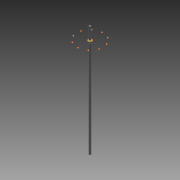
# Autodesk Inventor part: Worm Gear
Saved by Autodesk Inventor 2011 (Build 150239000, 239)
## iProperties
Created: 2011-11-28
Part Number: Worm Gear
Material: Steel, Mild
Document SubType Name: Modeling
Designer: Tom
Categories: <?xml version="1.0" encoding="UTF-16"?> <MemberInstance><Categories><FamilyTemplate><FamilyTemplateParameter ValueType="xs:double" Id="1" ObjectReferenceKey="da_z" ObjectType="kUserParameterObject"/><FamilyTemplateParameter ValueType="xs:double" Id="2" ObjectReferenceKey="da_b" ObjectType="kUserParameterObject"/><FamilyTemplateParameter ValueType="xs:double" Id="3" ObjectReferenceKey="da_beta" ObjectType="kUserParameterObject"/><FamilyTemplateParameter ValueType="xs:double" Id="4" ObjectReferenceKey="da_m" ObjectType="kUserParameterObject"/><FamilyTemplateParameter ValueType="xs:double" Id="5" ObjectReferenceKey="da_alpha" ObjectType="kUserParameterObject"/><FamilyTemplateParameter ValueType="xs:double" Id="6" ObjectReferenceKey="da_da" ObjectType="kUserParameterObject"/><FamilyTemplateParameter ValueType="xs:double" Id="7" ObjectReferenceKey="da_aw" ObjectType="kUserParameterObject"/><FamilyTemplateParameter ValueType="xs:double" Id="8" ObjectReferenceKey="da_px" ObjectType="kUserParameterObject"/><FamilyTemplateParameter ValueType="xs:double" Id="9" ObjectReferenceKey="da_d" ObjectType="kUserParameterObject"/><FamilyTemplateParameter ValueType="xs:double" Id="10" ObjectReferenceKey="da_dae" ObjectType="kUserParameterObject"/><FamilyTemplateParameter ValueType="xs:double" Id="11" ObjectReferenceKey="da_fi" ObjectType="kUserParameterObject"/><FamilyTemplateParameter ValueType="xs:string" Id="12" ObjectReferenceKey="EAIAABAAAAAWFwAAAAAAAIAAAAAAAAAA" ObjectType="83910656" SubObjectId="SurfaceGeometry"/></FamilyTemplate><ParamToTemplateMap><ParamToTemplate CategoryParameter="//CategoryParameter[@InternalName='046C89C9-8512-4d59-83FE-43B91F4F132A']" TemplateParameter="1"/><ParamToTemplate CategoryParameter="//CategoryParameter[@InternalName='2552DF32-E462-4b46-AEBF-C6C7768E72AC']" TemplateParameter="2"/><ParamToTemplate CategoryParameter="//CategoryParameter[@InternalName='C9EE641D-15FC-4fae-A226-E94C4372FDD7']" TemplateParameter="3"/><ParamToTemplate><ParamToTemplate CategoryParameter="//CategoryParameter[@InternalName='00B6519A-459B-49c7-AD84-2E56D39A5744']" ConstantValue="0.000000"/></ParamToTemplate><ParamToTemplate><ParamToTemplate CategoryParameter="//CategoryParameter[@InternalName='04B31F0E-C7A6-4894-AA32-9629BEFACF47']" ConstantValue="1.000000"/></ParamToTemplate><ParamToTemplate><ParamToTemplate CategoryParameter="//CategoryParameter[@InternalName='43CBEC2E-7847-49e7-A936-2F7889FCB2D9']" ConstantValue="0.200000"/></ParamToTemplate><ParamToTemplate><ParamToTemplate CategoryParameter="//CategoryParameter[@InternalName='B1EFC894-105D-4ebd-86BF-FA20ED196853']" ConstantValue="0.300000"/></ParamToTemplate><ParamToTemplate><ParamToTemplate CategoryParameter="//CategoryParameter[@InternalName='51175063-3D10-4879-93E8-6246FE8B403D']" ConstantValue="2060000000.000000"/></ParamToTemplate><ParamToTemplate><ParamToTemplate CategoryParameter="//CategoryParameter[@InternalName='A3A52E27-4454-46a9-B0BD-C932399B70AF']" ConstantValue="0.300000"/></ParamToTemplate><ParamToTemplate CategoryParameter="//CategoryParameter[@InternalName='91B76062-C214-41d9-B1B9-14D2AB99603D']" TemplateParameter="4"/><ParamToTemplate CategoryParameter="//CategoryParameter[@InternalName='2D373A89-B862-43d6-8D0B-0CBF12AB9F6C']" TemplateParameter="5"/><ParamToTemplate CategoryParameter="//CategoryParameter[@InternalName='37777632-D6A2-4fac-9D53-DB8ACD95C989']" TemplateParameter="6"/><ParamToTemplate CategoryParameter="//CategoryParameter[@InternalName='FD1017F1-B727-4f7e-9707-0F86F1FF9423']" TemplateParameter="7"/><ParamToTemplate CategoryParameter="//CategoryParameter[@InternalName='3BF567DA-17EF-48d8-80EA-D119B07F6463']" TemplateParameter="8"/><ParamToTemplate CategoryParameter="//CategoryParameter[@InternalName='BF5A1E7E-5373-4a22-AAD3-F583781FCF3C']" TemplateParameter="9"/><ParamToTemplate CategoryParameter="//CategoryParameter[@InternalName='2A200944-5A8C-41ca-B96E-8520D2E510F1']" TemplateParameter="10"/><ParamToTemplate CategoryParameter="//CategoryParameter[@InternalName='E77AC4FD-7B43-4566-B0ED-7CA70B976BC8']" TemplateParameter="11"/><ParamToTemplate><ParamToTemplate CategoryParameter="//CategoryParameter[@InternalName='D4F72237-D604-435a-AD0B-F738B7463A00']" ConstantValue="110.000000"/></ParamToTemplate><ParamToTemplate><ParamToTemplate CategoryParameter="//CategoryParameter[@InternalName='9E1B4470-B2D3-4ff1-B813-535BB4CDF51A']" ConstantValue="2000000.000000"/></ParamToTemplate><ParamToTemplate><ParamToTemplate CategoryParameter="//CategoryParameter[@InternalName='A7A89E9A-52E6-4d4f-86CF-A81914F22AA4']" ConstantValue="250000000.000000"/></ParamToTemplate><ParamToTemplate><ParamToTemplate CategoryParameter="//CategoryParameter[@InternalName='B02FABAC-469F-4ad8-A219-DB4578299DF6']" ConstantValue="250000000.000000"/></ParamToTemplate><ParamToTemplate><ParamToTemplate CategoryParameter="//CategoryParameter[@InternalName='E6981962-40D5-4343-A0AD-C263FCC47E10']" ConstantValue="9.000000"/></ParamToTemplate><ParamToTemplate><ParamToTemplate CategoryParameter="//CategoryParameter[@InternalName='B958E99F-2BCD-4955-8634-793EB7B37B89']" ConstantValue="8.000000"/></ParamToTemplate><ParamToTemplate><ParamToTemplate CategoryParameter="//CategoryParameter[@InternalName='4AD49A87-569D-440f-A541-E3B52A6A9DCE']" ConstantValue="1200.000000"/></ParamToTemplate><ParamToTemplate><ParamToTemplate CategoryParameter="//CategoryParameter[@InternalName='4E5813A0-330D-4b41-BE23-D880B01A1D55']" ConstantValue="1650000.000000"/></ParamToTemplate><ParamToTemplate><ParamToTemplate CategoryParameter="//CategoryParameter[@InternalName='19EB8C86-AA88-4253-B4AA-2F5DF1CE171A']" ConstantValue="6000.000000"/></ParamToTemplate><ParamToTemplate CategoryParameter="//CategoryParameter[@InternalName='27C3BAF2-7550-4e4b-AE2C-0DB134B7D9B7']" TemplateParameter="12"/></ParamToTemplateMap><Category DisplayName="Gear" InternalName="DC85795E-93AB-48d5-8EEE-5A27447B64BD" Mnemonic="Gear"><CategoryParameter DisplayName="z" InternalName="046C89C9-8512-4d59-83FE-43B91F4F132A" Mnemonic="z"/><CategoryParameter DisplayName="b|.2|" InternalName="2552DF32-E462-4b46-AEBF-C6C7768E72AC" Mnemonic="b"/><CategoryParameter DisplayName="||b|" InternalName="C9EE641D-15FC-4fae-A226-E94C4372FDD7" Mnemonic="beta"/><CategoryParameter DisplayName="x" InternalName="00B6519A-459B-49c7-AD84-2E56D39A5744" Mnemonic="x"/><CategoryParameter DisplayName="a*" InternalName="04B31F0E-C7A6-4894-AA32-9629BEFACF47" Mnemonic="a"/><CategoryParameter DisplayName="c*" InternalName="43CBEC2E-7847-49e7-A936-2F7889FCB2D9" Mnemonic="c"/><CategoryParameter DisplayName="r|.f|*" InternalName="B1EFC894-105D-4ebd-86BF-FA20ED196853" Mnemonic="rf"/><CategoryParameter DisplayName="E" InternalName="51175063-3D10-4879-93E8-6246FE8B403D" Mnemonic="E"/><CategoryParameter DisplayName="||m|" InternalName="A3A52E27-4454-46a9-B0BD-C932399B70AF" Mnemonic="mi"/><Category DisplayName="WormGear" InternalName="1B25C7EF-093B-4025-B3D3-619CD2A4550C" Mnemonic="WormGear"><CategoryParameter DisplayName="m" InternalName="91B76062-C214-41d9-B1B9-14D2AB99603D" Mnemonic="m"/><CategoryParameter DisplayName="||a|" InternalName="2D373A89-B862-43d6-8D0B-0CBF12AB9F6C" Mnemonic="alpha"/><CategoryParameter DisplayName="d|.a|" InternalName="37777632-D6A2-4fac-9D53-DB8ACD95C989" Mnemonic="da"/><CategoryParameter DisplayName="a|.w|" InternalName="FD1017F1-B727-4f7e-9707-0F86F1FF9423" Mnemonic="aw"/><CategoryParameter DisplayName="p|.x|" InternalName="3BF567DA-17EF-48d8-80EA-D119B07F6463" Mnemonic="px"/><CategoryParameter DisplayName="d" InternalName="BF5A1E7E-5373-4a22-AAD3-F583781FCF3C" Mnemonic="d"/><CategoryParameter DisplayName="dae" InternalName="2A200944-5A8C-41ca-B96E-8520D2E510F1" Mnemonic="dae"/><CategoryParameter DisplayName="||d|" InternalName="E77AC4FD-7B43-4566-B0ED-7CA70B976BC8" Mnemonic="fi"/><CategoryParameter DisplayName="VHV" InternalName="D4F72237-D604-435a-AD0B-F738B7463A00" Mnemonic="VHV"/><CategoryParameter DisplayName="||s||.Hlim|" InternalName="9E1B4470-B2D3-4ff1-B813-535BB4CDF51A" Mnemonic="sHlim"/><CategoryParameter DisplayName="N|.Flim|" InternalName="A7A89E9A-52E6-4d4f-86CF-A81914F22AA4" Mnemonic="NFlim"/><CategoryParameter DisplayName="N|.Hlim|" InternalName="B02FABAC-469F-4ad8-A219-DB4578299DF6" Mnemonic="NHlim"/><CategoryParameter DisplayName="q|.F|" InternalName="E6981962-40D5-4343-A0AD-C263FCC47E10" Mnemonic="qF"/><CategoryParameter DisplayName="q|.H|" InternalName="B958E99F-2BCD-4955-8634-793EB7B37B89" Mnemonic="qH"/><CategoryParameter DisplayName="v|.max|" InternalName="4AD49A87-569D-440f-A541-E3B52A6A9DCE" Mnemonic="maxv"/><CategoryParameter DisplayName="S|.n|" InternalName="4E5813A0-330D-4b41-BE23-D880B01A1D55" Mnemonic="Sn"/><CategoryParameter DisplayName="K|.w|" InternalName="19EB8C86-AA88-4253-B4AA-2F5DF1CE171A" Mnemonic="Kw"/><CategoryParameter DisplayName="PitchDiameter" InternalName="27C3BAF2-7550-4e4b-AE2C-0DB134B7D9B7" Mnemonic="IDS_PITCHDIAM"/></Category></Category></Categories></MemberInstance>
Density: 7.86 g/cm^3
Mass: 3.03532 g
Surface Area: 8.02106 cm^2
Volume: 0.386173 cm^3
CustomPartVersion: 1
Author: Tom
Autodesk Inventor part; units mm, degrees
ref_plane "Tooth Plane" through (0, -10, 0) normal (-0.0995037, 0, 0.9950372) x (0, 1, 0)
sketch "Base Body Sketch" plane through (0, 0, 0) normal (1, 0, 0) x (0, 1, 0)
  line L0 (0, -5.9034) -> (0, 5.9034) projected
  line L1 (0, 1.3) -> (1.8182, 1.3)
  line L2 (1.8182, 1.3) -> (2.1811, 0.9931)
  line L3 (-47.6302, 0) -> (47.6302, 0) construction
  circle A0 centre (3.3556, 0) radius 1.3422
  line L4 (2.1811, 0.9931) -> (2.1811, -0.9931)
  line L5 (0, -1.3) -> (1.8182, -1.3)
  line L6 (0, 1.3) -> (0, -1.3)
  line L7 (1.8182, -1.3) -> (2.1811, -0.9931)
  dimension "d50" = 40.218
  dimension "d87" = 4.3623
  dimension "d89" = 2.6845
  dimension "d92" = 2.6
  dimension "d93" = 3.3556
  constraints: 14 end point, 3 symmetric about line, 2 perpendicular, 2 point on line, 1 centre point, 1 collinear
  measures "d50" angle of L2 L1
  measures "d87" diameter of L4 L0
  measures "d89" diameter of A0
  measures "d92" distance of L1.start L5.start
  measures "d93" distance from line of A0.centre L6
revolve "Base Body" add sketch "Base Body Sketch" angle 360 about axis through (0, 0, 0) along (0, 0, 1) picked at (2.1456, -0.1336) contours L0 L1 L2 L4 A0 L7 L5 | A0 L4
revolve "Base Body2" cut sketch "Base Body Sketch" angle 360 about axis through (0, 0, 0) along (0, 0, 1) contours L4 A0 | A0 L4
sketch "Sketch8" plane through (0, 0, 1.3) normal (0, 0, 1) x (1, 0, 0)
  circle A0 centre (0, 0) radius 1.8182 projected
  circle A1 centre (0, 0) radius 1.6778
  dimension "d77" = 3.3556
  constraints: 1 centre point, 1 coincident
  measures "d77" diameter of A1
surface extrude "Pitch Diameter" sketch "Sketch8" against normal blind 2.6 shown no curves A1
ref_plane "Work Plane13" through (0, 0, 0) normal (-0.309017, 0.9510565, 0) x (0, 0, 1)
sketch "Tooth Sketch" plane through (0, -10, 0) normal (-0.0995037, 0, 0.9950372) x (0, 1, 0)
  line L0 (10, 48.2911) -> (10, -48.5255) projected
  line L1 (-37.6302, 0) -> (57.6302, 0) projected
  line L2 (6.6444, 0.4628) -> (6.6444, -0.4628)
  line L3 (6.6444, -0.4628) -> (7.9195, -0.4628)
  line L4 (7.9195, -0.4628) -> (8.7249, -0.1697)
  line L5 (8.7249, -0.1697) -> (8.7249, 0)
  line L6 (8.7249, 0.1697) -> (7.9195, 0.4628)
  line L7 (7.9195, 0.4628) -> (6.6444, 0.4628)
  line L8 (8.7249, 0.1697) -> (8.7249, 0)
  line L9 (8.3222, 0) -> (8.3222, -0.3163) construction
  dimension "d38" = 3.3556
  dimension "d39" = 20
  dimension "d40" = 1.2751
  dimension "d41" = 1.6778
  dimension "d42" = 0.3163
  constraints: 16 end point, 4 perpendicular, 3 equal length, 2 point on line, 1 midpoint, 1 parallel, 1 vertical
  measures "d38" distance between parallel lines of L0 L2
  measures "d39" angle of L6 L7
  measures "d40" distance of L6.end L2.start
  measures "d41" distance between parallel lines of L2 L9
  measures "d42" distance of L9.start L9.end
revolve "Tooth" cut sketch "Tooth Sketch" angle 360 about axis through (-0.4605, -3.3556, -0.0461) along (0.9950372, 0, 0.0995037)
pattern_circular "Tooth Pattern" count 10 over 360 about axis through (0, 0, 0) along (0, 0, 1) of "Tooth"
ref_plane "Work Plane14" through (0, 0, 0) normal (0.9510565, 0.309017, 0) x (0, 0, 1)
ref_plane "Work Plane15" through (0, 0, 0) normal (0, -1, 0) x (0, 0, 1)
sketch "Sketch10" plane through (0, 0, -1.3) normal (0, 0, -1) x (-0.7675295, -0.6410136, 0)
  arc A0 (1.2167, -1.3511) -> (1.6609, -0.7397) centre (0, 0) ccw projected
  circle A1 centre (0, 0) radius 1
  dimension "d97" = 2
  constraints: 1 centre point, 1 coincident
  measures "d97" diameter of A1
extrude "Extrusion2" add sketch "Sketch10" along normal blind 101.804
sketch "Sketch11" plane through (0, 0, 1.3) normal (0, 0, 1) x (0.928048, -0.3724605, 0)
  circle A0 centre (0, 0) radius 1 projected
  circle A1 centre (0, 0) radius 1
  constraints: 1 centre point, 1 coincident
sketch "Sketch12" plane through (0, 0, 1.3) normal (0, 0, 1) x (0.928048, -0.3724605, 0)
  arc A0 (-0.7397, -1.6609) -> (-0.7188, -1.624) centre (-0.7188, -1.624) ccw projected
  ellipse E0 centre (11.7872, -6.4282) end of major axis (32.0627, -11.5333) minor radius 2.0805 (-0.3814, -1.6807) -> (-0.7188, -1.624) ccw projected
  arc A1 (-0.3814, -1.6807) -> (-0.3778, -1.7785) centre (-0.3778, -1.7785) ccw projected
  arc A2 (-0.3778, -1.7785) -> (0.3778, -1.7785) centre (0, 0) ccw projected
  arc A3 (0.3778, -1.7785) -> (0.373, -1.7363) centre (0.373, -1.7363) ccw projected
  ellipse E1 centre (13.3144, 1.7279) end of major axis (32.7184, 9.5154) minor radius 2.0805 (0.6794, -1.5839) -> (0.373, -1.7363) ccw projected
  arc A4 (0.6794, -1.5839) -> (0.7397, -1.6609) centre (0.7397, -1.6609) ccw projected
  arc A5 (0.7397, -1.6609) -> (1.3511, -1.2167) centre (0, 0) ccw projected
  arc A6 (1.3511, -1.2167) -> (1.3224, -1.1855) centre (1.3224, -1.1855) ccw projected
  ellipse E2 centre (9.756, 9.2239) end of major axis (20.8767, 26.9295) minor radius 2.0805 (1.4806, -0.8821) -> (1.3224, -1.1855) ccw projected
  arc A7 (1.4806, -0.8821) -> (1.5747, -0.9089) centre (1.5747, -0.9089) ccw projected
  arc A8 (1.5747, -0.9089) -> (1.8082, -0.1902) centre (0, 0) ccw projected
  arc A9 (1.8082, -0.1902) -> (1.7666, -0.1818) centre (1.7666, -0.1818) ccw projected
  ellipse E3 centre (2.4711, 13.1967) end of major axis (1.0609, 34.0574) minor radius 2.0805 (1.7163, 0.1567) -> (1.7666, -0.1818) ccw projected
  arc A10 (1.7163, 0.1567) -> (1.8082, 0.1902) centre (1.8082, 0.1902) ccw projected
  arc A11 (1.8082, 0.1902) -> (1.5747, 0.9089) centre (0, 0) ccw projected
  arc A12 (1.5747, 0.9089) -> (1.5361, 0.8913) centre (1.5361, 0.8913) ccw projected
  ellipse E4 centre (-5.7577, 12.1289) end of major axis (-19.1602, 28.1766) minor radius 2.0805 (1.2964, 1.1356) -> (1.5361, 0.8913) ccw projected
  arc A13 (1.2964, 1.1356) -> (1.3511, 1.2167) centre (1.3511, 1.2167) ccw projected
  arc A14 (1.3511, 1.2167) -> (0.7397, 1.6609) centre (0, 0) ccw projected
  arc A15 (0.7397, 1.6609) -> (0.7188, 1.624) centre (0.7188, 1.624) ccw projected
  ellipse E5 centre (-11.7872, 6.4282) end of major axis (-32.0627, 11.5333) minor radius 2.0805 (0.3814, 1.6807) -> (0.7188, 1.624) ccw projected
  arc A16 (0.3814, 1.6807) -> (0.3778, 1.7785) centre (0.3778, 1.7785) ccw projected
  arc A17 (0.3778, 1.7785) -> (-0.3778, 1.7785) centre (0, 0) ccw projected
  arc A18 (-0.3778, 1.7785) -> (-0.373, 1.7363) centre (-0.373, 1.7363) ccw projected
  ellipse E6 centre (-13.3144, -1.7279) end of major axis (-32.7184, -9.5154) minor radius 2.0805 (-0.6794, 1.5839) -> (-0.373, 1.7363) ccw projected
  arc A19 (-0.6794, 1.5839) -> (-0.7397, 1.6609) centre (-0.7397, 1.6609) ccw projected
  arc A20 (-0.7397, 1.6609) -> (-1.3511, 1.2167) centre (0, 0) ccw projected
  arc A21 (-1.3511, 1.2167) -> (-1.3224, 1.1855) centre (-1.3224, 1.1855) ccw projected
  ellipse E7 centre (-9.756, -9.2239) end of major axis (-20.8767, -26.9295) minor radius 2.0805 (-1.4806, 0.8821) -> (-1.3224, 1.1855) ccw projected
  arc A22 (-1.4806, 0.8821) -> (-1.5747, 0.9089) centre (-1.5747, 0.9089) ccw projected
  arc A23 (-1.5747, 0.9089) -> (-1.8082, 0.1902) centre (0, 0) ccw projected
  arc A24 (-1.8082, 0.1902) -> (-1.7666, 0.1818) centre (-1.7666, 0.1818) ccw projected
  ellipse E8 centre (-2.4711, -13.1967) end of major axis (-1.0609, -34.0574) minor radius 2.0805 (-1.7163, -0.1567) -> (-1.7666, 0.1818) ccw projected
  arc A25 (-1.7163, -0.1567) -> (-1.8082, -0.1902) centre (-1.8082, -0.1902) ccw projected
  arc A26 (-1.8082, -0.1902) -> (-1.5747, -0.9089) centre (0, 0) ccw projected
  arc A27 (-1.5747, -0.9089) -> (-1.5361, -0.8913) centre (-1.5361, -0.8913) ccw projected
  ellipse E9 centre (5.7577, -12.1289) end of major axis (19.1602, -28.1766) minor radius 2.0805 (-1.2964, -1.1356) -> (-1.5361, -0.8913) ccw projected
  arc A28 (-1.2964, -1.1356) -> (-1.3511, -1.2167) centre (-1.3511, -1.2167) ccw projected
  arc A29 (-1.3511, -1.2167) -> (-0.7397, -1.6609) centre (0, 0) ccw projected
  circle A30 centre (0, 0) radius 1
  constraints: 1 centre point, 1 coincident, 30 other
extrude "Extrusion3" add sketch "Sketch11" along normal blind 12.938
equation "\"d50\" = da_fi"
equation "\"d87\" = da_dae"
equation "\"d89\" = 2 * da_aw - da_da"
equation "\"d92\" = da_b"
equation "\"d93\" = da_aw"
equation "\"d77\" = da_dw"
equation "\"d78\" = da_b"
equation "\"d38\" = da_aw"
equation "\"d39\" = da_alfat"
equation "\"d40\" = 0.5 * da_df1"
equation "\"d41\" = 0.5 * da_d1"
equation "\"d42\" = 0.3 * da_px"
equation "\"da_aw\" = 3.35558"
equation "\"da_fi\" = 40.2175deg"
equation "\"da_b\" = 2.6"
equation "\"da_df\" = 2.55024"
equation "\"da_da\" = 4.02669"
equation "\"da_beta\" = 5.710593deg"
equation "\"da_alfat\" = 20deg"
equation "\"da_df1\" = 2.55024"
equation "\"da_da1\" = 4.02669"
equation "\"da_d1\" = 3.35558"
equation "\"da_px\" = 1.05419"
equation "\"d68\" = da_aw"
equation "\"da_dw\" = 3.35558"
equation "\"da_rightdir\" = 0"
equation "\"d86\" = da_aw"
equation "\"da_dae\" = 4.36225"
body "Srf1"
body "Solid1"
